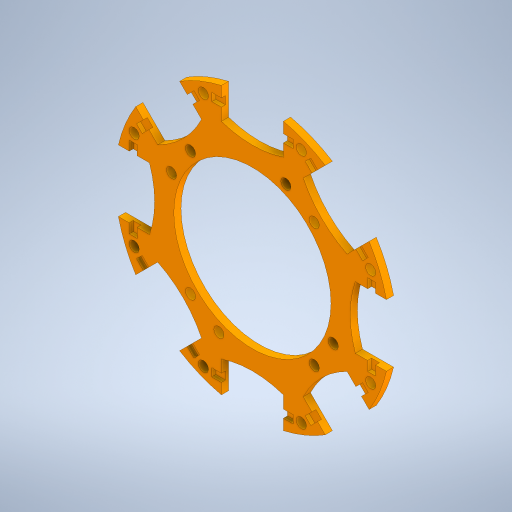
# Autodesk Inventor part: wheel_body_front
Saved by Autodesk Inventor 2024.1 (Build 281209000, 209)
## iProperties
Created: 2024-11-26
Part Number: wheel_body_front
Material: 一般
Document SubType Name: Modeling
Designer: hibik
Density: 1 g/cm^3
Appearance: 既定
Author: hibik
Autodesk Inventor part; units mm, degrees
ref_plane "YZ Plane" through (0, 0, 0) normal (1, 0, 0) x (0, 1, 0)
ref_plane "XZ Plane" through (0, 0, 0) normal (0, 1, 0) x (-1, 0, 0)
ref_plane "XY Plane" through (0, 0, 0) normal (0, 0, 1) x (1, 0, 0)
sketch "スケッチ1" plane through (0, 0, 0) normal (0, 0, 1) x (1, 0, 0)
  arc A0 (-9.75, 33.3881) -> (9.75, 33.3881) centre (0, 60.7) ccw
  arc A1 (-9.75, 32.3286) -> (9.75, 32.3286) centre (0, 60.7) ccw
  line L0 (-9.75, 57.7) -> (9.75, 57.7)
  line L1 (9.75, 57.7) -> (9.75, 30.7)
  line L2 (9.75, 30.7) -> (-9.75, 30.7)
  line L3 (-9.75, 30.7) -> (-9.75, 57.7)
  line L4 (-9.75, 44.7) -> (9.75, 44.7)
  circle A2 centre (0, 0) radius 23.7 construction
  circle A3 centre (0, 0) radius 24.7
  circle A4 centre (0, 0) radius 30.7 construction
  circle A5 centre (0, 0) radius 44.7
  line L5 (-28.6025, 14.8139) -> (-47.6944, 33.9058)
  arc A6 (-29.754, 15.9655) -> (-15.9655, 29.754) centre (-42.9214, 42.9214) ccw
  line L6 (-33.9058, 47.6944) -> (-14.8139, 28.6025)
  line L7 (-30.7, -9.75) -> (-57.7, -9.75)
  arc A7 (-32.3286, -9.75) -> (-32.3286, 9.75) centre (-60.7, 0) ccw
  line L8 (-57.7, 9.75) -> (-30.7, 9.75)
  line L9 (-14.8139, -28.6025) -> (-33.9058, -47.6944)
  arc A8 (-15.9655, -29.754) -> (-29.754, -15.9655) centre (-42.9214, -42.9214) ccw
  line L10 (-47.6944, -33.9058) -> (-28.6025, -14.8139)
  line L11 (9.75, -30.7) -> (9.75, -57.7)
  arc A9 (9.75, -32.3286) -> (-9.75, -32.3286) centre (0, -60.7) ccw
  line L12 (-9.75, -57.7) -> (-9.75, -30.7)
  line L13 (28.6025, -14.8139) -> (47.6944, -33.9058)
  arc A10 (29.754, -15.9655) -> (15.9655, -29.754) centre (42.9214, -42.9214) ccw
  line L14 (33.9058, -47.6944) -> (14.8139, -28.6025)
  line L15 (30.7, 9.75) -> (57.7, 9.75)
  arc A11 (32.3286, 9.75) -> (32.3286, -9.75) centre (60.7, 0) ccw
  line L16 (57.7, -9.75) -> (30.7, -9.75)
  line L17 (14.8139, 28.6025) -> (33.9058, 47.6944)
  arc A12 (15.9655, 29.754) -> (29.754, 15.9655) centre (42.9214, 42.9214) ccw
  line L18 (47.6944, 33.9058) -> (28.6025, 14.8139)
  circle A13 centre (0, 0) radius 43.2
  point P0 (0, 57.7)
  point P1 (-30.5033, 16.7147)
  point P2 (-24.7134, 38.502)
  point P3 (-16.7147, 30.5033)
  point P4 (-33.3881, -9.75)
  point P5 (-44.7, 9.75)
  point P6 (-33.3881, 9.75)
  point P7 (-16.7147, -30.5033)
  point P8 (-38.502, -24.7134)
  point P9 (-30.5033, -16.7147)
  point P10 (9.75, -33.3881)
  point P11 (-9.75, -44.7)
  point P12 (-9.75, -33.3881)
  point P13 (30.5033, -16.7147)
  point P14 (24.7134, -38.502)
  point P15 (16.7147, -30.5033)
  point P16 (33.3881, 9.75)
  point P17 (44.7, -9.75)
  point P18 (33.3881, -9.75)
  point P19 (16.7147, 30.5033)
  point P20 (38.502, 24.7134)
  point P21 (30.5033, 16.7147)
  point P22 (36.6531, -22.8646)
  point P23 (42.0854, -9.75)
  point P24 (42.0854, 9.75)
  point P25 (36.6531, 22.8646)
  point P26 (22.8646, 36.6531)
  point P27 (9.75, 42.0854)
  point P28 (-9.75, 42.0854)
  point P29 (-22.8646, 36.6531)
  point P30 (-36.6531, 22.8646)
  point P31 (-42.0854, 9.75)
  point P32 (-42.0854, -9.75)
  point P33 (-36.6531, -22.8646)
  point P34 (-22.8646, -36.6531)
  point P35 (-9.75, -42.0854)
  point P36 (9.75, -42.0854)
  point P37 (22.8646, -36.6531)
  point P38 (0, 30.7)
  dimension "d2" = 14
  dimension "d3" = 13
  dimension "d4" = 19.5
  dimension "d7" = 47.4
  dimension "d8" = 1
  dimension "d9" = 29
  dimension "d10" = 1
  dimension "d13" = 6
  dimension "d16" = 360
  dimension "d18" = 1.5
  dimension "d108" = 14
  dimension "d109" = 6
  constraints: 40 point on line, 38 end point, 18 point on circle, 14 centre point, 8 coincident, 3 tangent, 2 parallel, 2 perpendicular, 2 vertical alignment, 1 concentric, 1 horizontal, 1 midpoint, 105 other
  measures "d2" distance between parallel lines of L2 L4
  measures "d3" distance between parallel lines of L0 L4
  measures "d4" distance of L0.start L0.end
  measures "d7" diameter of A2
  measures "d8" radial gap between concentric circles of A3 A2
  measures "d9" radius of A0
  measures "d10" radial gap between concentric circles of A0 A1
  measures "d13" radial gap between concentric circles of A4 A3
  measures "d18" radial gap between concentric circles of A5 A13
  measures "d108" radial gap between concentric circles of A5 A4
  measures "d109" radial gap between concentric circles of A4 A3
extrude "押し出し1" add sketch "スケッチ1" along normal blind 2.25 contours L3 L2 L1 A13 L17 A12 L18 L15 A11 L16 L13 A10 L14 L11 A9 L12 L9 A8 L10 L7 A7 L8 L5 A6 L6 | A1 L2 L3 | L1 L2 A1
sketch "スケッチ2" plane through (0, 0, 2.25) normal (0, 0, 1) x (1, 0, 0)
  circle A0 centre (-15.3839, 37.14) radius 1.6
  line L0 (-15.3839, 37.14) -> (0, 0) construction
  line L1 (-9.75, 32.3286) -> (-9.75, 42.0854) projected
  line L2 (-22.8646, 36.6531) -> (-15.9655, 29.754) projected
  circle A1 centre (0, 0) radius 40.2 construction
  circle A2 centre (0, 0) radius 43.2 construction
  arc A3 (-9.75, 42.0854) -> (9.75, 42.0854) centre (0, 0) ccw projected
  circle A4 centre (-10.5238, 25.4067) radius 1.6
  line L3 (-10.5238, 25.4067) -> (-13.2002, 24.2981)
  circle A5 centre (0, 0) radius 24.7 projected
  circle A6 centre (-28.4257, 28.4257) radius 1.6
  circle A7 centre (-19.4454, 19.4454) radius 1.6
  circle A8 centre (-37.14, 15.3839) radius 1.6
  circle A9 centre (-25.4067, 10.5238) radius 1.6
  circle A10 centre (-40.2, 0) radius 1.6
  circle A11 centre (-27.5, 0) radius 1.6
  circle A12 centre (-37.14, -15.3839) radius 1.6
  circle A13 centre (-25.4067, -10.5238) radius 1.6
  circle A14 centre (-28.4257, -28.4257) radius 1.6
  circle A15 centre (-19.4454, -19.4454) radius 1.6
  circle A16 centre (-15.3839, -37.14) radius 1.6
  circle A17 centre (-10.5238, -25.4067) radius 1.6
  circle A18 centre (0, -40.2) radius 1.6
  circle A19 centre (0, -27.5) radius 1.6
  circle A20 centre (15.3839, -37.14) radius 1.6
  circle A21 centre (10.5238, -25.4067) radius 1.6
  circle A22 centre (28.4257, -28.4257) radius 1.6
  circle A23 centre (19.4454, -19.4454) radius 1.6
  circle A24 centre (37.14, -15.3839) radius 1.6
  circle A25 centre (25.4067, -10.5238) radius 1.6
  circle A26 centre (40.2, 0) radius 1.6
  circle A27 centre (27.5, 0) radius 1.6
  circle A28 centre (37.14, 15.3839) radius 1.6
  circle A29 centre (25.4067, 10.5238) radius 1.6
  circle A30 centre (28.4257, 28.4257) radius 1.6
  circle A31 centre (19.4454, 19.4454) radius 1.6
  circle A32 centre (15.3839, 37.14) radius 1.6
  circle A33 centre (10.5238, 25.4067) radius 1.6
  circle A34 centre (0, 40.2) radius 1.6
  circle A35 centre (0, 27.5) radius 1.6
  point P0 (-9.75, 57.7)
  point P1 (-9.75, 33.3881)
  dimension "d25" = 3
  dimension "d21" = 3.2
  dimension "d22" = 22.5
  dimension "d23" = 22.5
  dimension "d32" = 27.5
  dimension "d34" = 49.4
  dimension "d37" = 360
  constraints: 32 centre point, 4 end point, 2 coincident, 1 equal radius, 1 line through centre, 1 perpendicular, 1 point on line, 71 other
  measures "d21" diameter of A0
  measures "d22" angle of L1 L0
  measures "d23" angle of L2 L0
  measures "d32" distance from line of A5.centre L3
  measures "d34" diameter of A5
extrude "押し出し2" cut sketch "スケッチ2" against normal through all contours A0 | A7 | A8 | A9 | A12 | A15 | A16 | A17 | A20 | A23 | A24 | A25 | A28 | A31 | A32 | A33
sketch "スケッチ3" plane through (0, 0, 2.25) normal (0, 0, 1) x (1, 0, 0)
  line L0 (-9.75, 36.2017) -> (-12.75, 36.2017)
  line L1 (-12.75, 36.2017) -> (-12.75, 38.7017)
  line L2 (-12.75, 38.7017) -> (-9.75, 38.7017)
  line L3 (-9.75, 38.7017) -> (-9.75, 36.2017)
  line L4 (9.75, 36.2017) -> (12.75, 36.2017)
  line L5 (12.75, 36.2017) -> (12.75, 38.7017)
  line L6 (12.75, 38.7017) -> (9.75, 38.7017)
  line L7 (9.75, 38.7017) -> (9.75, 36.2017)
  line L8 (-32.4927, 18.7042) -> (-34.6141, 16.5828)
  line L9 (-34.6141, 16.5828) -> (-36.3818, 18.3506)
  line L10 (-36.3818, 18.3506) -> (-34.2605, 20.4719)
  line L11 (-34.2605, 20.4719) -> (-32.4927, 18.7042)
  line L12 (-20.4719, 34.2605) -> (-18.7042, 32.4927)
  line L13 (-18.7042, 32.4927) -> (-16.5828, 34.6141)
  line L14 (-16.5828, 34.6141) -> (-18.3506, 36.3818)
  line L15 (-18.3506, 36.3818) -> (-20.4719, 34.2605)
  line L16 (-36.2017, -9.75) -> (-36.2017, -12.75)
  line L17 (-36.2017, -12.75) -> (-38.7017, -12.75)
  line L18 (-38.7017, -12.75) -> (-38.7017, -9.75)
  line L19 (-38.7017, -9.75) -> (-36.2017, -9.75)
  line L20 (-38.7017, 9.75) -> (-36.2017, 9.75)
  line L21 (-36.2017, 9.75) -> (-36.2017, 12.75)
  line L22 (-36.2017, 12.75) -> (-38.7017, 12.75)
  line L23 (-38.7017, 12.75) -> (-38.7017, 9.75)
  line L24 (-18.7042, -32.4927) -> (-16.5828, -34.6141)
  line L25 (-16.5828, -34.6141) -> (-18.3506, -36.3818)
  line L26 (-18.3506, -36.3818) -> (-20.4719, -34.2605)
  line L27 (-20.4719, -34.2605) -> (-18.7042, -32.4927)
  line L28 (-34.2605, -20.4719) -> (-32.4927, -18.7042)
  line L29 (-32.4927, -18.7042) -> (-34.6141, -16.5828)
  line L30 (-34.6141, -16.5828) -> (-36.3818, -18.3506)
  line L31 (-36.3818, -18.3506) -> (-34.2605, -20.4719)
  line L32 (9.75, -36.2017) -> (12.75, -36.2017)
  line L33 (12.75, -36.2017) -> (12.75, -38.7017)
  line L34 (12.75, -38.7017) -> (9.75, -38.7017)
  line L35 (9.75, -38.7017) -> (9.75, -36.2017)
  line L36 (-9.75, -38.7017) -> (-9.75, -36.2017)
  line L37 (-9.75, -36.2017) -> (-12.75, -36.2017)
  line L38 (-12.75, -36.2017) -> (-12.75, -38.7017)
  line L39 (-12.75, -38.7017) -> (-9.75, -38.7017)
  line L40 (32.4927, -18.7042) -> (34.6141, -16.5828)
  line L41 (34.6141, -16.5828) -> (36.3818, -18.3506)
  line L42 (36.3818, -18.3506) -> (34.2605, -20.4719)
  line L43 (34.2605, -20.4719) -> (32.4927, -18.7042)
  line L44 (20.4719, -34.2605) -> (18.7042, -32.4927)
  line L45 (18.7042, -32.4927) -> (16.5828, -34.6141)
  line L46 (16.5828, -34.6141) -> (18.3506, -36.3818)
  line L47 (18.3506, -36.3818) -> (20.4719, -34.2605)
  line L48 (36.2017, 9.75) -> (36.2017, 12.75)
  line L49 (36.2017, 12.75) -> (38.7017, 12.75)
  line L50 (38.7017, 12.75) -> (38.7017, 9.75)
  line L51 (38.7017, 9.75) -> (36.2017, 9.75)
  line L52 (38.7017, -9.75) -> (36.2017, -9.75)
  line L53 (36.2017, -9.75) -> (36.2017, -12.75)
  line L54 (36.2017, -12.75) -> (38.7017, -12.75)
  line L55 (38.7017, -12.75) -> (38.7017, -9.75)
  line L56 (18.7042, 32.4927) -> (16.5828, 34.6141)
  line L57 (16.5828, 34.6141) -> (18.3506, 36.3818)
  line L58 (18.3506, 36.3818) -> (20.4719, 34.2605)
  line L59 (20.4719, 34.2605) -> (18.7042, 32.4927)
  line L60 (34.2605, 20.4719) -> (32.4927, 18.7042)
  line L61 (32.4927, 18.7042) -> (34.6141, 16.5828)
  line L62 (34.6141, 16.5828) -> (36.3818, 18.3506)
  line L63 (36.3818, 18.3506) -> (34.2605, 20.4719)
  line L64 (-9.75, 32.3286) -> (-9.75, 42.0854) projected
  line L65 (9.75, 42.0854) -> (9.75, 32.3286) projected
  circle A0 centre (-15.3839, 37.14) radius 1.6 projected
  circle A1 centre (0, 0) radius 38.7
  circle A2 centre (0, 0) radius 24.7 projected
  point P0 (-9.75, 37.4517)
  point P1 (-33.3766, 19.588)
  point P2 (-37.4517, -9.75)
  point P3 (-19.588, -33.3766)
  point P4 (9.75, -37.4517)
  point P5 (33.3766, -19.588)
  point P6 (37.4517, 9.75)
  point P7 (19.588, 33.3766)
  point P8 (-9.75, 33.3881)
  point P9 (9.75, 33.3881)
  point P10 (9.75, 37.4517)
  dimension "d40" = 2.5
  dimension "d45" = 360
  dimension "d105" = 3
  dimension "d107" = 14
  constraints: 128 end point, 16 point on line, 4 parallel, 3 collinear, 2 horizontal, 2 midpoint, 2 perpendicular, 1 coincident, 1 horizontal alignment, 140 other
  measures "d40" distance of L0.end L1.end
  measures "d105" distance of L1.end L2.end
extrude "押し出し3" cut sketch "スケッチ3" against normal blind 1.25 contours L0 L1 A1 L3 | A1 L1 L2 L3 | A1 L5 L4 L7 | L7 L6 L5 A1 | A1 L59 L56 L57 | L57 L58 L59 A1 | A1 L12 L15 L14 | L14 L13 L12 A1 | A1 L62 L61 L60 | L60 L63 L62 A1 | A1 L9 L10 L11 | L11 L8 L9 A1 | A1 L51 L48 L49 | L49 L50 L51 A1 | A1 L20 L23 L22 | L22 L21 L20 A1 | A1 L17 L18 L19 | L19 L16 L17 A1 | A1 L54 L53 L52 | L52 L55 L54 A1 | A1 L28 L31 L30 | L30 L29 L28 A1 | A1 L43 L40 L41 | L41 L42 L43 A1 | A1 L25 L26 L27 | L27 L24 L25 A1 | A1 L46 L45 L44 | L44 L47 L46 A1 | A1 L36 L39 L38 | L38 L37 L36 A1 | A1 L35 L32 L33 | L33 L34 L35 A1
equation "\"d22\" = d23"
